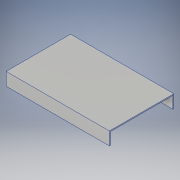
# Autodesk Inventor part: Spacer Extrusion
Saved by Autodesk Inventor 2019.4 (Build 234330000, 330)
## iProperties
Created: 2019-10-20
Part Number: Spacer Extrusion
Material: Aluminum 6061
Document SubType Name: Modeling
Designer: admin
Density: 2.7 g/cm^3
Appearance: Aluminum - Flat
Author: admin
Autodesk Inventor part; units mm, degrees
ref_plane "YZ Plane" through (0, 0, 0) normal (1, 0, 0) x (0, 1, 0)
ref_plane "XZ Plane" through (0, 0, 0) normal (0, 1, 0) x (-1, 0, 0)
ref_plane "XY Plane" through (0, 0, 0) normal (0, 0, 1) x (1, 0, 0)
sketch "Sketch1" plane through (0, 0, 0) normal (1, 0, 0) x (0, 1, 0)
  line L0 (0, 0) -> (25, 0)
  line L1 (25, 0) -> (25, -125)
  line L2 (25, -125) -> (0, -125)
  line L3 (0, -125) -> (0, -123)
  line L4 (0, -123) -> (23, -123)
  line L5 (23, -123) -> (23, -2)
  line L6 (23, -2) -> (0, -2)
  line L7 (0, -2) -> (0, 0)
  dimension "d0" = 2
  dimension "d1" = 2
  dimension "d2" = 125
  dimension "d3" = 25
  dimension "d4" = 2
  constraints: 16 end point, 7 perpendicular, 1 horizontal, 1 point on line
  measures "d0" distance of L6.end L0.start
  measures "d1" distance of L2.end L3.end
  measures "d2" distance of L0.end L1.end
  measures "d3" distance of L0.start L0.end
  measures "d4" distance between parallel lines of L1 L5
extrude "Extrusion1" add sketch "Sketch1" along normal blind 200
body "Solid1"
